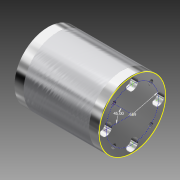
# Autodesk Inventor part: MOT_Gearbox_am0939
Saved by Autodesk Inventor 2013 (Build 170138000, 138)
## iProperties
Created: 2012-12-11
Part Number: MOT_Gearbox_am0939
Material: Steel, Mild
Document SubType Name: Modeling
Designer: Phillip
Density: 1 g/cm^3
Author: Phillip
Autodesk Inventor part; units mm, degrees
ref_plane "YZ Plane" through (0, 0, 0) normal (1, 0, 0) x (0, 1, 0)
ref_plane "XZ Plane" through (0, 0, 0) normal (0, 1, 0) x (-1, 0, 0)
ref_plane "XY Plane" through (0, 0, 0) normal (0, 0, 1) x (1, 0, 0)
sketch "Sketch1" plane through (0, 0, 0) normal (0, 0, 1) x (1, 0, 0)
  line L0 (0, 0) -> (0, 22.5044)
  line L1 (0, 22.5044) -> (6.35, 22.5044)
  line L2 (6.35, 22.5044) -> (6.35, 19.9644)
  line L3 (6.35, 19.9644) -> (50.165, 19.9644)
  line L4 (50.165, 19.9644) -> (50.165, 22.5044)
  line L5 (50.165, 22.5044) -> (56.515, 22.5044)
  line L6 (56.515, 22.5044) -> (56.515, 0)
  line L7 (0, 0) -> (56.515, 0)
  dimension "d0" = 22.5044
  dimension "d1" = 6.35
  dimension "d2" = 2.54
  dimension "d3" = 43.815
  dimension "d4" = 6.35
  constraints: 16 end point, 4 parallel, 2 perpendicular, 1 collinear, 1 vertical
  measures "d0" distance of L0.start L0.end
  measures "d1" distance of L0.end L1.end
  measures "d2" distance of L1.end L2.end
  measures "d3" distance of L2.end L3.end
  measures "d4" distance of L4.end L5.end
revolve "Revolution1" add sketch "Sketch1" angle 360 about axis through (0, 0, 0) along (1, 0, 0)
sketch "Sketch2" plane through (0, 0, 0) normal (0, 0, 1) x (1, 0, 0)
  line L0 (6.35, 19.9644) -> (50.165, 19.9644) projected
  line L1 (6.35, -22.5044) -> (6.35, 22.5044) projected
  line L2 (50.165, -22.5044) -> (50.165, 22.5044) projected
  line L3 (6.3525, 22.5044) -> (50.1625, 22.5044)
  line L4 (6.3525, 22.5044) -> (6.3525, 19.9644)
  line L5 (50.1625, 22.5044) -> (50.1625, 19.9644)
  line L6 (-11.303, 0) -> (67.818, 0) projected
  point P0 (0, 0)
  dimension "d6" = 0.0025
  dimension "d7" = 0.0025
  constraints: 6 end point, 3 perpendicular, 2 point on line
  measures "d6" distance between parallel lines of L2 L5
  measures "d7" distance between parallel lines of L1 L4
revolve "Revolution2" add sketch "Sketch2" angle 360 about axis through (-10, 0, 0) along (1, 0, 0) contours L4 L3 L5 L0
chamfer "Chamfer1" distance 0.254 angle 45 2 edges at (56.515, -22.5044, 0) (0, -22.5044, 0)
sketch "Sketch3" plane through (56.515, 0, 0) normal (1, 0, 0) x (0, 0, -1)
  circle A0 centre (0, 0) radius 22.2504 projected
  circle A1 centre (0, 0) radius 17.5006 construction
  line L0 (0, 0) -> (-12.3748, 12.3748) construction
  line L1 (0, 0) -> (-17.5006, 0) construction
  point P0 (0, 17.5006)
  point P1 (0, -17.5006)
  point P2 (17.5006, 0)
  dimension "d12" = 17.5006
  dimension "d14" = 45
  constraints: 5 point on circle, 4 end point, 1 centre point, 1 coincident, 1 horizontal
  measures "d12" radius of A1
  measures "d14" angle of L0 L1
hole "Hole1" at (56.515, 17.5006, 0) at (56.515, -17.5006, 0) at (56.515, 0, 17.5006) at (56.515, 0, -17.5006) direction (-1, 0, 0) diameter 4.4958 end through all counterbore diameter 8.001 counterbore depth 4.5974 clearance for "Socket Head Cap Screw ISO 4762" size "M4" standard "ISO"
hole "Hole2" at (56.515, 12.3748, 12.3748) direction (-1, 0, 0) diameter 3.2512 depth 9 tip angle 118
pattern_circular "Circular Pattern1" count 4 over 360 about axis through (-10, 0, 0) along (1, 0, 0) of "Hole2"
equation "\"d7\" = d6"
body "Solid1"
